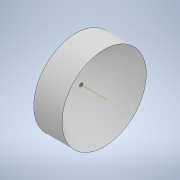
# Autodesk Inventor part: 2022plateForBall
Saved by Autodesk Inventor 2022.2 (Build 262287000, 287)
## iProperties
Created: 2020-01-14
Part Number: 2022plateForBall
Material: Generic
Document SubType Name: Modeling
Designer: steele
Density: 1 g/cm^3
Appearance: Default
Author: steele
Autodesk Inventor part; units mm, degrees
ref_plane "YZ Plane" through (0, 0, 0) normal (1, 0, 0) x (0, 1, 0)
ref_plane "XZ Plane" through (0, 0, 0) normal (0, 1, 0) x (-1, 0, 0)
ref_plane "XY Plane" through (0, 0, 0) normal (0, 0, 1) x (1, 0, 0)
sketch "Sketch4" plane through (0, 0, 0) normal (0, 0, 1) x (1, 0, 0)
  line L0 (0, 0) -> (101.6, 0) construction
  arc A0 (68.2819, 101.6) -> (12.7, 0) centre (133.35, 0) ccw
  line L1 (12.7, 0) -> (12.7, 96.7762) construction
  line L2 (0, 0) -> (0, 101.6)
  line L3 (0, 101.6) -> (68.2819, 101.6)
  line L4 (0, 0) -> (12.7, 0)
  dimension "d11" = 101.6
  dimension "d12" = 12.7
  dimension "d13" = 101.6
  dimension "d14" = 241.3
  constraints: 10 end point, 2 point on circle, 2 point on line, 2 vertical, 1 centre point, 1 collinear, 1 horizontal, 1 perpendicular, 1 tangent
  measures "d11" distance of L0.start L0.end
  measures "d12" distance from line of L0.start L1
  measures "d13" distance of L0.start L2.end
  measures "d14" diameter of A0
revolve "Revolution2" add sketch "Sketch4" angle 360 about axis through (0, 0, 0) along (1, 0, 0)
sketch "Sketch6" plane through (0, 0, 0) normal (-1, 0, 0) x (0, 0, 1)
  point P0 (0, 0)
  point P1 (0, 0)
  constraints: 1 coincident
hole "Hole1" at (0, 0, 0) direction (1, 0, 0) diameter 7.9248 end through all
body "Solid3"
